Autodesk Fusion 360 part; units mm, degrees
(part 5 of 5)
sketch "Sketch7" plane through (0, 0, 13) normal (0, 0, -1) x (-1, 0, 0)
  line L0 (38.5, 121.5) -> (21.5, 121.5)
  line L1 (21.5, 121.5) -> (21.5, 138.5)
  line L2 (21.5, 138.5) -> (38.5, 138.5)
  line L3 (38.5, 138.5) -> (38.5, 121.5)
  line L4 (18.5, 121.5) -> (1.5, 121.5)
  line L5 (1.5, 121.5) -> (1.5, 138.5)
  line L6 (1.5, 138.5) -> (18.5, 138.5)
  line L7 (18.5, 138.5) -> (18.5, 121.5)
  line L8 (-1.5, 121.5) -> (-18.5, 121.5)
  line L9 (-18.5, 121.5) -> (-18.5, 138.5)
  line L10 (-18.5, 138.5) -> (-1.5, 138.5)
  line L11 (-1.5, 138.5) -> (-1.5, 121.5)
  line L12 (-21.5, 121.5) -> (-38.5, 121.5)
  line L13 (-38.5, 121.5) -> (-38.5, 138.5)
  line L14 (-38.5, 138.5) -> (-21.5, 138.5)
  line L15 (-21.5, 138.5) -> (-21.5, 121.5)
  line L16 (-41.5, 121.5) -> (-58.5, 121.5)
  line L17 (-58.5, 121.5) -> (-58.5, 138.5)
  line L18 (-58.5, 138.5) -> (-41.5, 138.5)
  line L19 (-41.5, 138.5) -> (-41.5, 121.5)
  line L20 (-61.5, 121.5) -> (-78.5, 121.5)
  line L21 (-78.5, 121.5) -> (-78.5, 138.5)
  line L22 (-78.5, 138.5) -> (-61.5, 138.5)
  line L23 (-61.5, 138.5) -> (-61.5, 121.5)
  line L24 (-81.5, 121.5) -> (-98.5, 121.5)
  line L25 (-98.5, 121.5) -> (-98.5, 138.5)
  line L26 (-98.5, 138.5) -> (-81.5, 138.5)
  line L27 (-81.5, 138.5) -> (-81.5, 121.5)
  line L28 (98.5, 141.5) -> (81.5, 141.5)
  line L29 (81.5, 141.5) -> (81.5, 158.5)
  line L30 (81.5, 158.5) -> (98.5, 158.5)
  line L31 (98.5, 158.5) -> (98.5, 141.5)
  line L32 (78.5, 141.5) -> (61.5, 141.5)
  line L33 (61.5, 141.5) -> (61.5, 158.5)
  line L34 (61.5, 158.5) -> (78.5, 158.5)
  line L35 (78.5, 158.5) -> (78.5, 141.5)
  line L36 (58.5, 141.5) -> (41.5, 141.5)
  line L37 (41.5, 141.5) -> (41.5, 158.5)
  line L38 (41.5, 158.5) -> (58.5, 158.5)
  line L39 (58.5, 158.5) -> (58.5, 141.5)
  line L40 (38.5, 141.5) -> (21.5, 141.5)
  line L41 (21.5, 141.5) -> (21.5, 158.5)
  line L42 (21.5, 158.5) -> (38.5, 158.5)
  line L43 (38.5, 158.5) -> (38.5, 141.5)
  line L44 (18.5, 141.5) -> (1.5, 141.5)
  line L45 (1.5, 141.5) -> (1.5, 158.5)
  line L46 (1.5, 158.5) -> (18.5, 158.5)
  line L47 (18.5, 158.5) -> (18.5, 141.5)
  line L48 (-1.5, 141.5) -> (-18.5, 141.5)
  line L49 (-18.5, 141.5) -> (-18.5, 158.5)
  line L50 (-18.5, 158.5) -> (-1.5, 158.5)
  line L51 (-1.5, 158.5) -> (-1.5, 141.5)
  line L52 (-21.5, 141.5) -> (-38.5, 141.5)
  line L53 (-38.5, 141.5) -> (-38.5, 158.5)
  line L54 (-38.5, 158.5) -> (-21.5, 158.5)
  line L55 (-21.5, 158.5) -> (-21.5, 141.5)
  line L56 (-41.5, 141.5) -> (-58.5, 141.5)
  line L57 (-58.5, 141.5) -> (-58.5, 158.5)
  line L58 (-58.5, 158.5) -> (-41.5, 158.5)
  line L59 (-41.5, 158.5) -> (-41.5, 141.5)
  line L60 (-61.5, 141.5) -> (-78.5, 141.5)
  line L61 (-78.5, 141.5) -> (-78.5, 158.5)
  line L62 (-78.5, 158.5) -> (-61.5, 158.5)
  line L63 (-61.5, 158.5) -> (-61.5, 141.5)
  line L64 (-81.5, 141.5) -> (-98.5, 141.5)
  line L65 (-98.5, 141.5) -> (-98.5, 158.5)
  line L66 (-98.5, 158.5) -> (-81.5, 158.5)
  line L67 (-81.5, 158.5) -> (-81.5, 141.5)
  line L68 (98.5, 161.5) -> (81.5, 161.5)
  line L69 (81.5, 161.5) -> (81.5, 178.5)
  line L70 (81.5, 178.5) -> (98.5, 178.5)
  line L71 (98.5, 178.5) -> (98.5, 161.5)
  line L72 (78.5, 161.5) -> (61.5, 161.5)
  line L73 (61.5, 161.5) -> (61.5, 178.5)
  line L74 (61.5, 178.5) -> (78.5, 178.5)
  line L75 (78.5, 178.5) -> (78.5, 161.5)
  line L76 (58.5, 161.5) -> (41.5, 161.5)
  line L77 (41.5, 161.5) -> (41.5, 178.5)
  line L78 (41.5, 178.5) -> (58.5, 178.5)
  line L79 (58.5, 178.5) -> (58.5, 161.5)
  line L80 (58.5, 121.5) -> (41.5, 121.5)
  line L81 (41.5, 121.5) -> (41.5, 138.5)
  line L82 (41.5, 138.5) -> (58.5, 138.5)
  line L83 (58.5, 138.5) -> (58.5, 121.5)
  line L84 (98.5, -98.5) -> (81.5, -98.5)
  line L85 (81.5, -98.5) -> (81.5, -81.5)
  line L86 (81.5, -81.5) -> (98.5, -81.5)
  line L87 (98.5, -81.5) -> (98.5, -98.5)
  line L88 (-1.5, -58.5) -> (-18.5, -58.5)
  line L89 (-18.5, -58.5) -> (-18.5, -41.5)
  line L90 (-18.5, -41.5) -> (-1.5, -41.5)
  line L91 (-1.5, -41.5) -> (-1.5, -58.5)
  line L92 (-81.5, -118.5) -> (-98.5, -118.5)
  line L93 (-98.5, -118.5) -> (-98.5, -101.5)
  line L94 (-98.5, -101.5) -> (-81.5, -101.5)
  line L95 (-81.5, -101.5) -> (-81.5, -118.5)
  line L96 (-61.5, -118.5) -> (-78.5, -118.5)
  line L97 (-78.5, -118.5) -> (-78.5, -101.5)
  line L98 (-78.5, -101.5) -> (-61.5, -101.5)
  line L99 (-61.5, -101.5) -> (-61.5, -118.5)
  line L100 (-41.5, -118.5) -> (-58.5, -118.5)
  line L101 (-58.5, -118.5) -> (-58.5, -101.5)
  line L102 (-58.5, -101.5) -> (-41.5, -101.5)
  line L103 (-41.5, -101.5) -> (-41.5, -118.5)
  line L104 (-21.5, -118.5) -> (-38.5, -118.5)
  line L105 (-38.5, -118.5) -> (-38.5, -101.5)
  line L106 (-38.5, -101.5) -> (-21.5, -101.5)
  line L107 (-21.5, -101.5) -> (-21.5, -118.5)
  line L108 (-1.5, -118.5) -> (-18.5, -118.5)
  line L109 (-18.5, -118.5) -> (-18.5, -101.5)
  line L110 (-18.5, -101.5) -> (-1.5, -101.5)
  line L111 (-1.5, -101.5) -> (-1.5, -118.5)
  line L112 (18.5, -118.5) -> (1.5, -118.5)
  line L113 (1.5, -118.5) -> (1.5, -101.5)
  line L114 (1.5, -101.5) -> (18.5, -101.5)
  line L115 (18.5, -101.5) -> (18.5, -118.5)
  line L116 (38.5, -118.5) -> (21.5, -118.5)
  line L117 (21.5, -118.5) -> (21.5, -101.5)
  line L118 (21.5, -101.5) -> (38.5, -101.5)
  line L119 (38.5, -101.5) -> (38.5, -118.5)
  line L120 (58.5, -118.5) -> (41.5, -118.5)
  line L121 (41.5, -118.5) -> (41.5, -101.5)
  line L122 (41.5, -101.5) -> (58.5, -101.5)
  line L123 (58.5, -101.5) -> (58.5, -118.5)
  line L124 (78.5, -118.5) -> (61.5, -118.5)
  line L125 (61.5, -118.5) -> (61.5, -101.5)
  line L126 (61.5, -101.5) -> (78.5, -101.5)
  line L127 (78.5, -101.5) -> (78.5, -118.5)
  line L128 (98.5, -118.5) -> (81.5, -118.5)
  line L129 (81.5, -118.5) -> (81.5, -101.5)
  line L130 (81.5, -101.5) -> (98.5, -101.5)
  line L131 (98.5, -101.5) -> (98.5, -118.5)
  line L132 (-81.5, -138.5) -> (-98.5, -138.5)
  line L133 (-98.5, -138.5) -> (-98.5, -121.5)
  line L134 (-98.5, -121.5) -> (-81.5, -121.5)
  line L135 (-81.5, -121.5) -> (-81.5, -138.5)
  line L136 (-61.5, -138.5) -> (-78.5, -138.5)
  line L137 (-78.5, -138.5) -> (-78.5, -121.5)
  line L138 (-78.5, -121.5) -> (-61.5, -121.5)
  line L139 (-61.5, -121.5) -> (-61.5, -138.5)
  line L140 (-41.5, -138.5) -> (-58.5, -138.5)
  line L141 (-58.5, -138.5) -> (-58.5, -121.5)
  line L142 (-58.5, -121.5) -> (-41.5, -121.5)
  line L143 (-41.5, -121.5) -> (-41.5, -138.5)
  line L144 (-21.5, -138.5) -> (-38.5, -138.5)
  line L145 (-38.5, -138.5) -> (-38.5, -121.5)
  line L146 (-38.5, -121.5) -> (-21.5, -121.5)
  line L147 (-21.5, -121.5) -> (-21.5, -138.5)
  line L148 (-1.5, -138.5) -> (-18.5, -138.5)
  line L149 (-18.5, -138.5) -> (-18.5, -121.5)
  line L150 (-18.5, -121.5) -> (-1.5, -121.5)
  line L151 (-1.5, -121.5) -> (-1.5, -138.5)
  line L152 (18.5, -138.5) -> (1.5, -138.5)
  line L153 (1.5, -138.5) -> (1.5, -121.5)
  line L154 (1.5, -121.5) -> (18.5, -121.5)
  line L155 (18.5, -121.5) -> (18.5, -138.5)
  line L156 (38.5, -138.5) -> (21.5, -138.5)
  line L157 (21.5, -138.5) -> (21.5, -121.5)
  line L158 (21.5, -121.5) -> (38.5, -121.5)
  line L159 (38.5, -121.5) -> (38.5, -138.5)
  line L160 (58.5, -138.5) -> (41.5, -138.5)
  line L161 (41.5, -138.5) -> (41.5, -121.5)
  line L162 (41.5, -121.5) -> (58.5, -121.5)
  line L163 (58.5, -121.5) -> (58.5, -138.5)
  line L164 (78.5, -138.5) -> (61.5, -138.5)
  line L165 (61.5, -138.5) -> (61.5, -121.5)
  line L166 (61.5, -121.5) -> (78.5, -121.5)
  line L167 (78.5, -121.5) -> (78.5, -138.5)
  line L168 (98.5, -138.5) -> (81.5, -138.5)
  line L169 (81.5, -138.5) -> (81.5, -121.5)
  line L170 (81.5, -121.5) -> (98.5, -121.5)
  line L171 (98.5, -121.5) -> (98.5, -138.5)
  line L172 (-81.5, -158.5) -> (-98.5, -158.5)
  line L173 (-98.5, -158.5) -> (-98.5, -141.5)
  line L174 (-98.5, -141.5) -> (-81.5, -141.5)
  line L175 (-81.5, -141.5) -> (-81.5, -158.5)
  line L176 (-61.5, -158.5) -> (-78.5, -158.5)
  line L177 (-78.5, -158.5) -> (-78.5, -141.5)
  line L178 (-78.5, -141.5) -> (-61.5, -141.5)
  line L179 (-61.5, -141.5) -> (-61.5, -158.5)
  line L180 (-41.5, -158.5) -> (-58.5, -158.5)
  line L181 (-58.5, -158.5) -> (-58.5, -141.5)
  line L182 (-58.5, -141.5) -> (-41.5, -141.5)
  line L183 (-41.5, -141.5) -> (-41.5, -158.5)
  line L184 (-21.5, -158.5) -> (-38.5, -158.5)
  line L185 (-38.5, -158.5) -> (-38.5, -141.5)
  line L186 (-38.5, -141.5) -> (-21.5, -141.5)
  line L187 (-21.5, -141.5) -> (-21.5, -158.5)
  line L188 (-1.5, -158.5) -> (-18.5, -158.5)
  line L189 (-18.5, -158.5) -> (-18.5, -141.5)
  line L190 (-18.5, -141.5) -> (-1.5, -141.5)
  line L191 (-1.5, -141.5) -> (-1.5, -158.5)
  line L192 (18.5, -158.5) -> (1.5, -158.5)
  line L193 (1.5, -158.5) -> (1.5, -141.5)
  line L194 (1.5, -141.5) -> (18.5, -141.5)
  line L195 (18.5, -141.5) -> (18.5, -158.5)
  line L196 (38.5, -158.5) -> (21.5, -158.5)
  line L197 (21.5, -158.5) -> (21.5, -141.5)
  line L198 (21.5, -141.5) -> (38.5, -141.5)
  line L199 (38.5, -141.5) -> (38.5, -158.5)
  line L200 (58.5, -158.5) -> (41.5, -158.5)
  line L201 (41.5, -158.5) -> (41.5, -141.5)
  line L202 (41.5, -141.5) -> (58.5, -141.5)
  line L203 (58.5, -141.5) -> (58.5, -158.5)
  line L204 (-41.5, -58.5) -> (-58.5, -58.5)
  line L205 (-58.5, -58.5) -> (-58.5, -41.5)
  line L206 (-58.5, -41.5) -> (-41.5, -41.5)
  line L207 (-41.5, -41.5) -> (-41.5, -58.5)
  line L208 (98.5, -201.5) -> (98.5, -218.5)
  line L209 (98.5, -218.5) -> (81.5, -218.5)
  line L210 (81.5, -218.5) -> (81.5, -201.5)
  line L211 (81.5, -201.5) -> (98.5, -201.5)
  line L212 (78.5, -218.5) -> (61.5, -218.5)
  line L213 (61.5, -218.5) -> (61.5, -201.5)
  line L214 (61.5, -201.5) -> (78.5, -201.5)
  line L215 (78.5, -201.5) -> (78.5, -218.5)
  line L216 (58.5, -218.5) -> (41.5, -218.5)
  line L217 (41.5, -218.5) -> (41.5, -201.5)
  line L218 (41.5, -201.5) -> (58.5, -201.5)
  line L219 (58.5, -201.5) -> (58.5, -218.5)
  line L220 (38.5, -218.5) -> (21.5, -218.5)
  line L221 (21.5, -218.5) -> (21.5, -201.5)
  line L222 (21.5, -201.5) -> (38.5, -201.5)
  line L223 (38.5, -201.5) -> (38.5, -218.5)
  line L224 (18.5, -218.5) -> (1.5, -218.5)
  line L225 (1.5, -218.5) -> (1.5, -201.5)
  line L226 (1.5, -201.5) -> (18.5, -201.5)
  line L227 (18.5, -201.5) -> (18.5, -218.5)
  line L228 (-1.5, -218.5) -> (-18.5, -218.5)
  line L229 (-18.5, -218.5) -> (-18.5, -201.5)
  line L230 (-18.5, -201.5) -> (-1.5, -201.5)
  line L231 (-1.5, -201.5) -> (-1.5, -218.5)
  line L232 (-21.5, -218.5) -> (-38.5, -218.5)
  line L233 (-38.5, -218.5) -> (-38.5, -201.5)
  line L234 (-38.5, -201.5) -> (-21.5, -201.5)
  line L235 (-21.5, -201.5) -> (-21.5, -218.5)
  line L236 (-41.5, -218.5) -> (-58.5, -218.5)
  line L237 (-58.5, -218.5) -> (-58.5, -201.5)
  line L238 (-58.5, -201.5) -> (-41.5, -201.5)
  line L239 (-41.5, -201.5) -> (-41.5, -218.5)
  line L240 (-61.5, -218.5) -> (-78.5, -218.5)
  line L241 (-78.5, -218.5) -> (-78.5, -201.5)
  line L242 (-78.5, -201.5) -> (-61.5, -201.5)
  line L243 (-61.5, -201.5) -> (-61.5, -218.5)
  line L244 (-81.5, -218.5) -> (-98.5, -218.5)
  line L245 (-98.5, -218.5) -> (-98.5, -201.5)
  line L246 (-98.5, -201.5) -> (-81.5, -201.5)
  line L247 (-81.5, -201.5) -> (-81.5, -218.5)
  line L248 (98.5, -198.5) -> (81.5, -198.5)
  line L249 (81.5, -198.5) -> (81.5, -181.5)
  line L250 (81.5, -181.5) -> (98.5, -181.5)
  line L251 (98.5, -181.5) -> (98.5, -198.5)
  line L252 (78.5, -198.5) -> (61.5, -198.5)
  line L253 (61.5, -198.5) -> (61.5, -181.5)
  line L254 (61.5, -181.5) -> (78.5, -181.5)
  line L255 (78.5, -181.5) -> (78.5, -198.5)
  line L256 (58.5, -198.5) -> (41.5, -198.5)
  line L257 (41.5, -198.5) -> (41.5, -181.5)
  line L258 (41.5, -181.5) -> (58.5, -181.5)
  line L259 (58.5, -181.5) -> (58.5, -198.5)
  line L260 (38.5, -198.5) -> (21.5, -198.5)
  line L261 (21.5, -198.5) -> (21.5, -181.5)
  line L262 (21.5, -181.5) -> (38.5, -181.5)
  line L263 (38.5, -181.5) -> (38.5, -198.5)
  line L264 (18.5, -198.5) -> (1.5, -198.5)
  line L265 (1.5, -198.5) -> (1.5, -181.5)
  line L266 (1.5, -181.5) -> (18.5, -181.5)
  line L267 (18.5, -181.5) -> (18.5, -198.5)
  line L268 (-1.5, -198.5) -> (-18.5, -198.5)
  line L269 (-18.5, -198.5) -> (-18.5, -181.5)
  line L270 (-18.5, -181.5) -> (-1.5, -181.5)
  line L271 (-1.5, -181.5) -> (-1.5, -198.5)
  line L272 (-21.5, -198.5) -> (-38.5, -198.5)
  line L273 (-38.5, -198.5) -> (-38.5, -181.5)
  line L274 (-38.5, -181.5) -> (-21.5, -181.5)
  line L275 (-21.5, -181.5) -> (-21.5, -198.5)
  line L276 (-41.5, -198.5) -> (-58.5, -198.5)
  line L277 (-58.5, -198.5) -> (-58.5, -181.5)
  line L278 (-58.5, -181.5) -> (-41.5, -181.5)
  line L279 (-41.5, -181.5) -> (-41.5, -198.5)
  line L280 (-61.5, -198.5) -> (-78.5, -198.5)
  line L281 (-78.5, -198.5) -> (-78.5, -181.5)
  line L282 (-78.5, -181.5) -> (-61.5, -181.5)
  line L283 (-61.5, -181.5) -> (-61.5, -198.5)
  line L284 (-81.5, -198.5) -> (-98.5, -198.5)
  line L285 (-98.5, -198.5) -> (-98.5, -181.5)
  line L286 (-98.5, -181.5) -> (-81.5, -181.5)
  line L287 (-81.5, -181.5) -> (-81.5, -198.5)
  line L288 (98.5, -178.5) -> (81.5, -178.5)
  line L289 (81.5, -178.5) -> (81.5, -161.5)
  line L290 (81.5, -161.5) -> (98.5, -161.5)
  line L291 (98.5, -161.5) -> (98.5, -178.5)
  line L292 (78.5, -178.5) -> (61.5, -178.5)
  line L293 (61.5, -178.5) -> (61.5, -161.5)
  line L294 (61.5, -161.5) -> (78.5, -161.5)
  line L295 (78.5, -161.5) -> (78.5, -178.5)
  line L296 (58.5, -178.5) -> (41.5, -178.5)
  line L297 (41.5, -178.5) -> (41.5, -161.5)
  line L298 (41.5, -161.5) -> (58.5, -161.5)
  line L299 (58.5, -161.5) -> (58.5, -178.5)
  line L300 (38.5, -178.5) -> (21.5, -178.5)
  line L301 (21.5, -178.5) -> (21.5, -161.5)
  line L302 (21.5, -161.5) -> (38.5, -161.5)
  line L303 (38.5, -161.5) -> (38.5, -178.5)
  line L304 (18.5, -178.5) -> (1.5, -178.5)
  line L305 (1.5, -178.5) -> (1.5, -161.5)
  line L306 (1.5, -161.5) -> (18.5, -161.5)
  line L307 (18.5, -161.5) -> (18.5, -178.5)
  line L308 (-1.5, -178.5) -> (-18.5, -178.5)
  line L309 (-18.5, -178.5) -> (-18.5, -161.5)
  line L310 (-18.5, -161.5) -> (-1.5, -161.5)
  line L311 (-1.5, -161.5) -> (-1.5, -178.5)
  line L312 (98.5, -158.5) -> (81.5, -158.5)
  line L313 (81.5, -158.5) -> (81.5, -141.5)
  line L314 (81.5, -141.5) -> (98.5, -141.5)
  line L315 (98.5, -141.5) -> (98.5, -158.5)
  line L316 (78.5, -158.5) -> (61.5, -158.5)
  line L317 (61.5, -158.5) -> (61.5, -141.5)
  line L318 (61.5, -141.5) -> (78.5, -141.5)
  line L319 (78.5, -141.5) -> (78.5, -158.5)
  line L320 (-81.5, -178.5) -> (-98.5, -178.5)
  line L321 (-98.5, -178.5) -> (-98.5, -161.5)
  line L322 (-98.5, -161.5) -> (-81.5, -161.5)
  line L323 (-81.5, -161.5) -> (-81.5, -178.5)
  line L324 (-61.5, -178.5) -> (-78.5, -178.5)
  line L325 (-78.5, -178.5) -> (-78.5, -161.5)
  line L326 (-78.5, -161.5) -> (-61.5, -161.5)
  line L327 (-61.5, -161.5) -> (-61.5, -178.5)
  line L328 (-41.5, -178.5) -> (-58.5, -178.5)
  line L329 (-58.5, -178.5) -> (-58.5, -161.5)
  line L330 (-58.5, -161.5) -> (-41.5, -161.5)
  line L331 (-41.5, -161.5) -> (-41.5, -178.5)
  line L332 (-21.5, -178.5) -> (-38.5, -178.5)
  line L333 (-38.5, -178.5) -> (-38.5, -161.5)
  line L334 (-38.5, -161.5) -> (-21.5, -161.5)
  line L335 (-21.5, -161.5) -> (-21.5, -178.5)
  line L336 (38.5, 161.5) -> (21.5, 161.5)
  line L337 (21.5, 161.5) -> (21.5, 178.5)
  line L338 (21.5, 178.5) -> (38.5, 178.5)
  line L339 (38.5, 178.5) -> (38.5, 161.5)
  line L340 (78.5, -98.5) -> (61.5, -98.5)
  line L341 (61.5, -98.5) -> (61.5, -81.5)
  line L342 (61.5, -81.5) -> (78.5, -81.5)
  line L343 (78.5, -81.5) -> (78.5, -98.5)
  line L344 (98.5, 121.5) -> (81.5, 121.5)
  line L345 (81.5, 121.5) -> (81.5, 138.5)
  line L346 (81.5, 138.5) -> (98.5, 138.5)
  line L347 (98.5, 138.5) -> (98.5, 121.5)
  line L348 (-81.5, 101.5) -> (-98.5, 101.5)
  line L349 (-98.5, 101.5) -> (-98.5, 118.5)
  line L350 (-98.5, 118.5) -> (-81.5, 118.5)
  line L351 (-81.5, 118.5) -> (-81.5, 101.5)
  line L352 (-61.5, 101.5) -> (-78.5, 101.5)
  line L353 (-78.5, 101.5) -> (-78.5, 118.5)
  line L354 (-78.5, 118.5) -> (-61.5, 118.5)
  line L355 (-61.5, 118.5) -> (-61.5, 101.5)
  line L356 (-41.5, 101.5) -> (-58.5, 101.5)
  line L357 (-58.5, 101.5) -> (-58.5, 118.5)
  line L358 (-58.5, 118.5) -> (-41.5, 118.5)
  line L359 (-41.5, 118.5) -> (-41.5, 101.5)
  line L360 (-21.5, 101.5) -> (-38.5, 101.5)
  line L361 (-38.5, 101.5) -> (-38.5, 118.5)
  line L362 (-38.5, 118.5) -> (-21.5, 118.5)
  line L363 (-21.5, 118.5) -> (-21.5, 101.5)
  line L364 (-1.5, 101.5) -> (-18.5, 101.5)
  line L365 (-18.5, 101.5) -> (-18.5, 118.5)
  line L366 (-18.5, 118.5) -> (-1.5, 118.5)
  line L367 (-1.5, 118.5) -> (-1.5, 101.5)
  line L368 (18.5, 101.5) -> (1.5, 101.5)
  line L369 (1.5, 101.5) -> (1.5, 118.5)
  line L370 (1.5, 118.5) -> (18.5, 118.5)
  line L371 (18.5, 118.5) -> (18.5, 101.5)
  line L372 (38.5, 101.5) -> (21.5, 101.5)
  line L373 (21.5, 101.5) -> (21.5, 118.5)
  line L374 (21.5, 118.5) -> (38.5, 118.5)
  line L375 (38.5, 118.5) -> (38.5, 101.5)
  line L376 (58.5, 101.5) -> (41.5, 101.5)
  line L377 (41.5, 101.5) -> (41.5, 118.5)
  line L378 (41.5, 118.5) -> (58.5, 118.5)
  line L379 (58.5, 118.5) -> (58.5, 101.5)
  line L380 (78.5, 101.5) -> (61.5, 101.5)
  line L381 (61.5, 101.5) -> (61.5, 118.5)
  line L382 (61.5, 118.5) -> (78.5, 118.5)
  line L383 (78.5, 118.5) -> (78.5, 101.5)
  line L384 (98.5, 101.5) -> (81.5, 101.5)
  line L385 (81.5, 101.5) -> (81.5, 118.5)
  line L386 (81.5, 118.5) -> (98.5, 118.5)
  line L387 (98.5, 118.5) -> (98.5, 101.5)
  line L388 (-81.5, 81.5) -> (-98.5, 81.5)
  line L389 (-98.5, 81.5) -> (-98.5, 98.5)
  line L390 (-98.5, 98.5) -> (-81.5, 98.5)
  line L391 (-81.5, 98.5) -> (-81.5, 81.5)
  line L392 (-61.5, 81.5) -> (-78.5, 81.5)
  line L393 (-78.5, 81.5) -> (-78.5, 98.5)
  line L394 (-78.5, 98.5) -> (-61.5, 98.5)
  line L395 (-61.5, 98.5) -> (-61.5, 81.5)
  line L396 (-41.5, 81.5) -> (-58.5, 81.5)
  line L397 (-58.5, 81.5) -> (-58.5, 98.5)
  line L398 (-58.5, 98.5) -> (-41.5, 98.5)
  line L399 (-41.5, 98.5) -> (-41.5, 81.5)
  line L400 (-21.5, 81.5) -> (-38.5, 81.5)
  line L401 (-38.5, 81.5) -> (-38.5, 98.5)
  line L402 (-38.5, 98.5) -> (-21.5, 98.5)
  line L403 (-21.5, 98.5) -> (-21.5, 81.5)
  line L404 (-1.5, 81.5) -> (-18.5, 81.5)
  line L405 (-18.5, 81.5) -> (-18.5, 98.5)
  line L406 (-18.5, 98.5) -> (-1.5, 98.5)
  line L407 (-1.5, 98.5) -> (-1.5, 81.5)
  line L408 (18.5, 81.5) -> (1.5, 81.5)
  line L409 (1.5, 81.5) -> (1.5, 98.5)
  line L410 (1.5, 98.5) -> (18.5, 98.5)
  line L411 (18.5, 98.5) -> (18.5, 81.5)
  line L412 (38.5, 81.5) -> (21.5, 81.5)
  line L413 (21.5, 81.5) -> (21.5, 98.5)
  line L414 (21.5, 98.5) -> (38.5, 98.5)
  line L415 (38.5, 98.5) -> (38.5, 81.5)
  line L416 (58.5, 81.5) -> (41.5, 81.5)
  line L417 (41.5, 81.5) -> (41.5, 98.5)
  line L418 (41.5, 98.5) -> (58.5, 98.5)
  line L419 (58.5, 98.5) -> (58.5, 81.5)
  line L420 (78.5, 81.5) -> (61.5, 81.5)
  line L421 (61.5, 81.5) -> (61.5, 98.5)
  line L422 (61.5, 98.5) -> (78.5, 98.5)
  line L423 (78.5, 98.5) -> (78.5, 81.5)
  line L424 (98.5, 81.5) -> (81.5, 81.5)
  line L425 (81.5, 81.5) -> (81.5, 98.5)
  line L426 (81.5, 98.5) -> (98.5, 98.5)
  line L427 (98.5, 98.5) -> (98.5, 81.5)
  line L428 (-81.5, 61.5) -> (-98.5, 61.5)
  line L429 (-98.5, 61.5) -> (-98.5, 78.5)
  line L430 (-98.5, 78.5) -> (-81.5, 78.5)
  line L431 (-81.5, 78.5) -> (-81.5, 61.5)
  line L432 (-61.5, 61.5) -> (-78.5, 61.5)
  line L433 (-78.5, 61.5) -> (-78.5, 78.5)
  line L434 (-78.5, 78.5) -> (-61.5, 78.5)
  line L435 (-61.5, 78.5) -> (-61.5, 61.5)
  line L436 (-41.5, 61.5) -> (-58.5, 61.5)
  line L437 (-58.5, 61.5) -> (-58.5, 78.5)
  line L438 (-58.5, 78.5) -> (-41.5, 78.5)
  line L439 (-41.5, 78.5) -> (-41.5, 61.5)
  line L440 (-21.5, 61.5) -> (-38.5, 61.5)
  line L441 (-38.5, 61.5) -> (-38.5, 78.5)
  line L442 (-38.5, 78.5) -> (-21.5, 78.5)
  line L443 (-21.5, 78.5) -> (-21.5, 61.5)
  line L444 (-1.5, 61.5) -> (-18.5, 61.5)
  line L445 (-18.5, 61.5) -> (-18.5, 78.5)
  line L446 (-18.5, 78.5) -> (-1.5, 78.5)
  line L447 (-1.5, 78.5) -> (-1.5, 61.5)
  line L448 (18.5, 61.5) -> (1.5, 61.5)
  line L449 (1.5, 61.5) -> (1.5, 78.5)
  line L450 (1.5, 78.5) -> (18.5, 78.5)
  line L451 (18.5, 78.5) -> (18.5, 61.5)
  line L452 (38.5, 61.5) -> (21.5, 61.5)
  line L453 (21.5, 61.5) -> (21.5, 78.5)
  line L454 (21.5, 78.5) -> (38.5, 78.5)
  line L455 (38.5, 78.5) -> (38.5, 61.5)
  line L456 (58.5, 61.5) -> (41.5, 61.5)
  line L457 (41.5, 61.5) -> (41.5, 78.5)
  line L458 (41.5, 78.5) -> (58.5, 78.5)
  line L459 (58.5, 78.5) -> (58.5, 61.5)
  line L460 (78.5, 61.5) -> (61.5, 61.5)
  line L461 (61.5, 61.5) -> (61.5, 78.5)
  line L462 (61.5, 78.5) -> (78.5, 78.5)
  line L463 (78.5, 78.5) -> (78.5, 61.5)
  line L464 (98.5, 61.5) -> (81.5, 61.5)
  line L465 (81.5, 61.5) -> (81.5, 78.5)
  line L466 (81.5, 78.5) -> (98.5, 78.5)
  line L467 (98.5, 78.5) -> (98.5, 61.5)
  line L468 (-81.5, 41.5) -> (-98.5, 41.5)
  line L469 (-98.5, 41.5) -> (-98.5, 58.5)
  line L470 (-98.5, 58.5) -> (-81.5, 58.5)
  line L471 (-81.5, 58.5) -> (-81.5, 41.5)
  line L472 (-61.5, 41.5) -> (-78.5, 41.5)
  line L473 (-78.5, 41.5) -> (-78.5, 58.5)
  line L474 (-78.5, 58.5) -> (-61.5, 58.5)
  line L475 (-61.5, 58.5) -> (-61.5, 41.5)
  line L476 (-41.5, 41.5) -> (-58.5, 41.5)
  line L477 (-58.5, 41.5) -> (-58.5, 58.5)
  line L478 (-58.5, 58.5) -> (-41.5, 58.5)
  line L479 (-41.5, 58.5) -> (-41.5, 41.5)
  line L480 (-21.5, 41.5) -> (-38.5, 41.5)
  line L481 (-38.5, 41.5) -> (-38.5, 58.5)
  line L482 (-38.5, 58.5) -> (-21.5, 58.5)
  line L483 (-21.5, 58.5) -> (-21.5, 41.5)
  line L484 (-1.5, 41.5) -> (-18.5, 41.5)
  line L485 (-18.5, 41.5) -> (-18.5, 58.5)
  line L486 (-18.5, 58.5) -> (-1.5, 58.5)
  line L487 (-1.5, 58.5) -> (-1.5, 41.5)
  line L488 (18.5, 41.5) -> (1.5, 41.5)
  line L489 (1.5, 41.5) -> (1.5, 58.5)
  line L490 (1.5, 58.5) -> (18.5, 58.5)
  line L491 (18.5, 58.5) -> (18.5, 41.5)
  line L492 (38.5, 41.5) -> (21.5, 41.5)
  line L493 (21.5, 41.5) -> (21.5, 58.5)
  line L494 (21.5, 58.5) -> (38.5, 58.5)
  line L495 (38.5, 58.5) -> (38.5, 41.5)
  line L496 (58.5, 41.5) -> (41.5, 41.5)
  line L497 (41.5, 41.5) -> (41.5, 58.5)
  line L498 (41.5, 58.5) -> (58.5, 58.5)
  line L499 (58.5, 58.5) -> (58.5, 41.5)
  line L500 (78.5, 41.5) -> (61.5, 41.5)
  line L501 (61.5, 41.5) -> (61.5, 58.5)
  line L502 (61.5, 58.5) -> (78.5, 58.5)
  line L503 (78.5, 58.5) -> (78.5, 41.5)
  line L504 (98.5, 41.5) -> (81.5, 41.5)
  line L505 (81.5, 41.5) -> (81.5, 58.5)
  line L506 (81.5, 58.5) -> (98.5, 58.5)
  line L507 (98.5, 58.5) -> (98.5, 41.5)
  line L508 (-81.5, 21.5) -> (-98.5, 21.5)
  line L509 (-98.5, 21.5) -> (-98.5, 38.5)
  line L510 (-98.5, 38.5) -> (-81.5, 38.5)
  line L511 (-81.5, 38.5) -> (-81.5, 21.5)
  line L512 (-61.5, 21.5) -> (-78.5, 21.5)
  line L513 (-78.5, 21.5) -> (-78.5, 38.5)
  line L514 (-78.5, 38.5) -> (-61.5, 38.5)
  line L515 (-61.5, 38.5) -> (-61.5, 21.5)
  line L516 (-41.5, 21.5) -> (-58.5, 21.5)
  line L517 (-58.5, 21.5) -> (-58.5, 38.5)
  line L518 (-58.5, 38.5) -> (-41.5, 38.5)
  line L519 (-41.5, 38.5) -> (-41.5, 21.5)
  line L520 (-21.5, 21.5) -> (-38.5, 21.5)
  line L521 (-38.5, 21.5) -> (-38.5, 38.5)
  line L522 (-38.5, 38.5) -> (-21.5, 38.5)
  line L523 (-21.5, 38.5) -> (-21.5, 21.5)
  line L524 (-1.5, 21.5) -> (-18.5, 21.5)
  line L525 (-18.5, 21.5) -> (-18.5, 38.5)
  line L526 (-18.5, 38.5) -> (-1.5, 38.5)
  line L527 (-1.5, 38.5) -> (-1.5, 21.5)
  line L528 (18.5, 21.5) -> (1.5, 21.5)
  line L529 (1.5, 21.5) -> (1.5, 38.5)
  line L530 (1.5, 38.5) -> (18.5, 38.5)
  line L531 (18.5, 38.5) -> (18.5, 21.5)
  line L532 (38.5, 21.5) -> (21.5, 21.5)
  line L533 (21.5, 21.5) -> (21.5, 38.5)
  line L534 (21.5, 38.5) -> (38.5, 38.5)
  line L535 (38.5, 38.5) -> (38.5, 21.5)
  line L536 (58.5, 21.5) -> (41.5, 21.5)
  line L537 (41.5, 21.5) -> (41.5, 38.5)
  line L538 (41.5, 38.5) -> (58.5, 38.5)
  line L539 (58.5, 38.5) -> (58.5, 21.5)
  line L540 (78.5, 21.5) -> (61.5, 21.5)
  line L541 (61.5, 21.5) -> (61.5, 38.5)
  line L542 (61.5, 38.5) -> (78.5, 38.5)
  line L543 (78.5, 38.5) -> (78.5, 21.5)
  line L544 (98.5, 21.5) -> (81.5, 21.5)
  line L545 (81.5, 21.5) -> (81.5, 38.5)
  line L546 (81.5, 38.5) -> (98.5, 38.5)
  line L547 (98.5, 38.5) -> (98.5, 21.5)
  line L548 (-81.5, 1.5) -> (-98.5, 1.5)
  line L549 (-98.5, 1.5) -> (-98.5, 18.5)
  line L550 (-98.5, 18.5) -> (-81.5, 18.5)
  line L551 (-81.5, 18.5) -> (-81.5, 1.5)
  line L552 (-61.5, 1.5) -> (-78.5, 1.5)
  line L553 (-78.5, 1.5) -> (-78.5, 18.5)
  line L554 (-78.5, 18.5) -> (-61.5, 18.5)
  line L555 (-61.5, 18.5) -> (-61.5, 1.5)
  line L556 (-41.5, 1.5) -> (-58.5, 1.5)
  line L557 (-58.5, 1.5) -> (-58.5, 18.5)
  line L558 (-58.5, 18.5) -> (-41.5, 18.5)
  line L559 (-41.5, 18.5) -> (-41.5, 1.5)
  line L560 (-21.5, 1.5) -> (-38.5, 1.5)
  line L561 (-38.5, 1.5) -> (-38.5, 18.5)
  line L562 (-38.5, 18.5) -> (-21.5, 18.5)
  line L563 (-21.5, 18.5) -> (-21.5, 1.5)
  line L564 (-1.5, 1.5) -> (-18.5, 1.5)
  line L565 (-18.5, 1.5) -> (-18.5, 18.5)
  line L566 (-18.5, 18.5) -> (-1.5, 18.5)
  line L567 (-1.5, 18.5) -> (-1.5, 1.5)
  line L568 (18.5, 1.5) -> (1.5, 1.5)
  line L569 (1.5, 1.5) -> (1.5, 18.5)
  line L570 (1.5, 18.5) -> (18.5, 18.5)
  line L571 (18.5, 18.5) -> (18.5, 1.5)
  line L572 (38.5, 1.5) -> (21.5, 1.5)
  line L573 (21.5, 1.5) -> (21.5, 18.5)
  line L574 (21.5, 18.5) -> (38.5, 18.5)
  line L575 (38.5, 18.5) -> (38.5, 1.5)
  line L576 (58.5, 1.5) -> (41.5, 1.5)
  line L577 (41.5, 1.5) -> (41.5, 18.5)
  line L578 (41.5, 18.5) -> (58.5, 18.5)
  line L579 (58.5, 18.5) -> (58.5, 1.5)
  line L580 (78.5, 1.5) -> (61.5, 1.5)
  line L581 (61.5, 1.5) -> (61.5, 18.5)
  line L582 (61.5, 18.5) -> (78.5, 18.5)
  line L583 (78.5, 18.5) -> (78.5, 1.5)
  line L584 (98.5, 1.5) -> (81.5, 1.5)
  line L585 (81.5, 1.5) -> (81.5, 18.5)
  line L586 (81.5, 18.5) -> (98.5, 18.5)
  line L587 (98.5, 18.5) -> (98.5, 1.5)
  line L588 (-81.5, -18.5) -> (-98.5, -18.5)
  line L589 (-98.5, -18.5) -> (-98.5, -1.5)
  line L590 (-98.5, -1.5) -> (-81.5, -1.5)
  line L591 (-81.5, -1.5) -> (-81.5, -18.5)
  line L592 (-61.5, -18.5) -> (-78.5, -18.5)
  line L593 (-78.5, -18.5) -> (-78.5, -1.5)
  line L594 (-78.5, -1.5) -> (-61.5, -1.5)
  line L595 (-61.5, -1.5) -> (-61.5, -18.5)
  line L596 (-41.5, -18.5) -> (-58.5, -18.5)
  line L597 (-58.5, -18.5) -> (-58.5, -1.5)
  line L598 (-58.5, -1.5) -> (-41.5, -1.5)
  line L599 (-41.5, -1.5) -> (-41.5, -18.5)
  line L600 (-21.5, -18.5) -> (-38.5, -18.5)
  line L601 (-38.5, -18.5) -> (-38.5, -1.5)
  line L602 (-38.5, -1.5) -> (-21.5, -1.5)
  line L603 (-21.5, -1.5) -> (-21.5, -18.5)
  line L604 (-1.5, -18.5) -> (-18.5, -18.5)
  line L605 (-18.5, -18.5) -> (-18.5, -1.5)
  line L606 (-18.5, -1.5) -> (-1.5, -1.5)
  line L607 (-1.5, -1.5) -> (-1.5, -18.5)
  line L608 (18.5, -18.5) -> (1.5, -18.5)
  line L609 (1.5, -18.5) -> (1.5, -1.5)
  line L610 (1.5, -1.5) -> (18.5, -1.5)
  line L611 (18.5, -1.5) -> (18.5, -18.5)
  line L612 (38.5, -18.5) -> (21.5, -18.5)
  line L613 (21.5, -18.5) -> (21.5, -1.5)
  line L614 (21.5, -1.5) -> (38.5, -1.5)
  line L615 (38.5, -1.5) -> (38.5, -18.5)
  line L616 (58.5, -18.5) -> (41.5, -18.5)
  line L617 (41.5, -18.5) -> (41.5, -1.5)
  line L618 (41.5, -1.5) -> (58.5, -1.5)
  line L619 (58.5, -1.5) -> (58.5, -18.5)
  line L620 (78.5, -18.5) -> (61.5, -18.5)
  line L621 (61.5, -18.5) -> (61.5, -1.5)
  line L622 (61.5, -1.5) -> (78.5, -1.5)
  line L623 (78.5, -1.5) -> (78.5, -18.5)
  line L624 (98.5, -18.5) -> (81.5, -18.5)
  line L625 (81.5, -18.5) -> (81.5, -1.5)
  line L626 (81.5, -1.5) -> (98.5, -1.5)
  line L627 (98.5, -1.5) -> (98.5, -18.5)
  line L628 (-81.5, -38.5) -> (-98.5, -38.5)
  line L629 (-98.5, -38.5) -> (-98.5, -21.5)
  line L630 (-98.5, -21.5) -> (-81.5, -21.5)
  line L631 (-81.5, -21.5) -> (-81.5, -38.5)
  line L632 (-61.5, -38.5) -> (-78.5, -38.5)
  line L633 (-78.5, -38.5) -> (-78.5, -21.5)
  line L634 (-78.5, -21.5) -> (-61.5, -21.5)
  line L635 (-61.5, -21.5) -> (-61.5, -38.5)
  line L636 (-41.5, -38.5) -> (-58.5, -38.5)
  line L637 (-58.5, -38.5) -> (-58.5, -21.5)
  line L638 (-58.5, -21.5) -> (-41.5, -21.5)
  line L639 (-41.5, -21.5) -> (-41.5, -38.5)
  line L640 (-21.5, -38.5) -> (-38.5, -38.5)
  line L641 (-38.5, -38.5) -> (-38.5, -21.5)
  line L642 (-38.5, -21.5) -> (-21.5, -21.5)
  line L643 (-21.5, -21.5) -> (-21.5, -38.5)
  line L644 (-1.5, -38.5) -> (-18.5, -38.5)
  line L645 (-18.5, -38.5) -> (-18.5, -21.5)
  line L646 (-18.5, -21.5) -> (-1.5, -21.5)
  line L647 (-1.5, -21.5) -> (-1.5, -38.5)
  line L648 (18.5, -38.5) -> (1.5, -38.5)
  line L649 (1.5, -38.5) -> (1.5, -21.5)
  line L650 (1.5, -21.5) -> (18.5, -21.5)
  line L651 (18.5, -21.5) -> (18.5, -38.5)
  line L652 (38.5, -38.5) -> (21.5, -38.5)
  line L653 (21.5, -38.5) -> (21.5, -21.5)
  line L654 (21.5, -21.5) -> (38.5, -21.5)
  line L655 (38.5, -21.5) -> (38.5, -38.5)
  line L656 (58.5, -38.5) -> (41.5, -38.5)
  line L657 (41.5, -38.5) -> (41.5, -21.5)
  line L658 (41.5, -21.5) -> (58.5, -21.5)
  line L659 (58.5, -21.5) -> (58.5, -38.5)
  line L660 (78.5, -38.5) -> (61.5, -38.5)
  line L661 (61.5, -38.5) -> (61.5, -21.5)
  line L662 (61.5, -21.5) -> (78.5, -21.5)
  line L663 (78.5, -21.5) -> (78.5, -38.5)
  line L664 (98.5, -38.5) -> (81.5, -38.5)
  line L665 (81.5, -38.5) -> (81.5, -21.5)
  line L666 (81.5, -21.5) -> (98.5, -21.5)
  line L667 (98.5, -21.5) -> (98.5, -38.5)
  line L668 (-81.5, -58.5) -> (-98.5, -58.5)
  line L669 (-98.5, -58.5) -> (-98.5, -41.5)
  line L670 (-98.5, -41.5) -> (-81.5, -41.5)
  line L671 (-81.5, -41.5) -> (-81.5, -58.5)
  line L672 (-61.5, -58.5) -> (-78.5, -58.5)
  line L673 (-78.5, -58.5) -> (-78.5, -41.5)
  line L674 (-78.5, -41.5) -> (-61.5, -41.5)
  line L675 (-61.5, -41.5) -> (-61.5, -58.5)
  line L676 (-81.5, 201.5) -> (-98.5, 201.5)
  line L677 (-98.5, 201.5) -> (-98.5, 218.5)
  line L678 (-98.5, 218.5) -> (-81.5, 218.5)
  line L679 (-81.5, 218.5) -> (-81.5, 201.5)
  line L680 (-61.5, 201.5) -> (-78.5, 201.5)
  line L681 (-78.5, 201.5) -> (-78.5, 218.5)
  line L682 (-78.5, 218.5) -> (-61.5, 218.5)
  line L683 (-61.5, 218.5) -> (-61.5, 201.5)
  line L684 (-41.5, 201.5) -> (-58.5, 201.5)
  line L685 (-58.5, 201.5) -> (-58.5, 218.5)
  line L686 (-58.5, 218.5) -> (-41.5, 218.5)
  line L687 (-41.5, 218.5) -> (-41.5, 201.5)
  line L688 (-21.5, 201.5) -> (-38.5, 201.5)
  line L689 (-38.5, 201.5) -> (-38.5, 218.5)
  line L690 (-38.5, 218.5) -> (-21.5, 218.5)
  line L691 (-21.5, 218.5) -> (-21.5, 201.5)
  line L692 (-1.5, 201.5) -> (-18.5, 201.5)
  line L693 (-18.5, 201.5) -> (-18.5, 218.5)
  line L694 (-18.5, 218.5) -> (-1.5, 218.5)
  line L695 (-1.5, 218.5) -> (-1.5, 201.5)
  line L696 (18.5, 201.5) -> (1.5, 201.5)
  line L697 (1.5, 201.5) -> (1.5, 218.5)
  line L698 (1.5, 218.5) -> (18.5, 218.5)
  line L699 (18.5, 218.5) -> (18.5, 201.5)
  line L700 (38.5, 201.5) -> (21.5, 201.5)
  line L701 (21.5, 201.5) -> (21.5, 218.5)
  line L702 (21.5, 218.5) -> (38.5, 218.5)
  line L703 (38.5, 218.5) -> (38.5, 201.5)
  line L704 (58.5, 201.5) -> (41.5, 201.5)
  line L705 (41.5, 201.5) -> (41.5, 218.5)
  line L706 (41.5, 218.5) -> (58.5, 218.5)
  line L707 (58.5, 218.5) -> (58.5, 201.5)
  line L708 (78.5, 201.5) -> (61.5, 201.5)
  line L709 (61.5, 201.5) -> (61.5, 218.5)
  line L710 (61.5, 218.5) -> (78.5, 218.5)
  line L711 (78.5, 218.5) -> (78.5, 201.5)
  line L712 (98.5, 201.5) -> (81.5, 201.5)
  line L713 (81.5, 201.5) -> (81.5, 218.5)
  line L714 (81.5, 218.5) -> (98.5, 218.5)
  line L715 (98.5, 218.5) -> (98.5, 201.5)
  line L716 (-81.5, 181.5) -> (-98.5, 181.5)
  line L717 (-98.5, 181.5) -> (-98.5, 198.5)
  line L718 (-98.5, 198.5) -> (-81.5, 198.5)
  line L719 (-81.5, 198.5) -> (-81.5, 181.5)
  line L720 (-61.5, 181.5) -> (-78.5, 181.5)
  line L721 (-78.5, 181.5) -> (-78.5, 198.5)
  line L722 (-78.5, 198.5) -> (-61.5, 198.5)
  line L723 (-61.5, 198.5) -> (-61.5, 181.5)
  line L724 (-41.5, 181.5) -> (-58.5, 181.5)
  line L725 (-58.5, 181.5) -> (-58.5, 198.5)
  line L726 (-58.5, 198.5) -> (-41.5, 198.5)
  line L727 (-41.5, 198.5) -> (-41.5, 181.5)
  line L728 (-21.5, 181.5) -> (-38.5, 181.5)
  line L729 (-38.5, 181.5) -> (-38.5, 198.5)
  line L730 (-38.5, 198.5) -> (-21.5, 198.5)
  line L731 (-21.5, 198.5) -> (-21.5, 181.5)
  line L732 (-1.5, 181.5) -> (-18.5, 181.5)
  line L733 (-18.5, 181.5) -> (-18.5, 198.5)
  line L734 (-18.5, 198.5) -> (-1.5, 198.5)
  line L735 (-1.5, 198.5) -> (-1.5, 181.5)
  line L736 (18.5, 181.5) -> (1.5, 181.5)
  line L737 (1.5, 181.5) -> (1.5, 198.5)
  line L738 (1.5, 198.5) -> (18.5, 198.5)
  line L739 (18.5, 198.5) -> (18.5, 181.5)
  line L740 (38.5, 181.5) -> (21.5, 181.5)
  line L741 (21.5, 181.5) -> (21.5, 198.5)
  line L742 (21.5, 198.5) -> (38.5, 198.5)
  line L743 (38.5, 198.5) -> (38.5, 181.5)
  line L744 (58.5, 181.5) -> (41.5, 181.5)
  line L745 (41.5, 181.5) -> (41.5, 198.5)
  line L746 (41.5, 198.5) -> (58.5, 198.5)
  line L747 (58.5, 198.5) -> (58.5, 181.5)
  line L748 (78.5, 181.5) -> (61.5, 181.5)
  line L749 (61.5, 181.5) -> (61.5, 198.5)
  line L750 (61.5, 198.5) -> (78.5, 198.5)
  line L751 (78.5, 198.5) -> (78.5, 181.5)
  line L752 (98.5, 181.5) -> (81.5, 181.5)
  line L753 (81.5, 181.5) -> (81.5, 198.5)
  line L754 (81.5, 198.5) -> (98.5, 198.5)
  line L755 (98.5, 198.5) -> (98.5, 181.5)
  line L756 (-81.5, 161.5) -> (-98.5, 161.5)
  line L757 (-98.5, 161.5) -> (-98.5, 178.5)
  line L758 (-98.5, 178.5) -> (-81.5, 178.5)
  line L759 (-81.5, 178.5) -> (-81.5, 161.5)
  line L760 (-61.5, 161.5) -> (-78.5, 161.5)
  line L761 (-78.5, 161.5) -> (-78.5, 178.5)
  line L762 (-78.5, 178.5) -> (-61.5, 178.5)
  line L763 (-61.5, 178.5) -> (-61.5, 161.5)
  line L764 (-41.5, 161.5) -> (-58.5, 161.5)
  line L765 (-58.5, 161.5) -> (-58.5, 178.5)
  line L766 (-58.5, 178.5) -> (-41.5, 178.5)
  line L767 (-41.5, 178.5) -> (-41.5, 161.5)
  line L768 (-21.5, 161.5) -> (-38.5, 161.5)
  line L769 (-38.5, 161.5) -> (-38.5, 178.5)
  line L770 (-38.5, 178.5) -> (-21.5, 178.5)
  line L771 (-21.5, 178.5) -> (-21.5, 161.5)
  line L772 (-1.5, 161.5) -> (-18.5, 161.5)
  line L773 (-18.5, 161.5) -> (-18.5, 178.5)
  line L774 (-18.5, 178.5) -> (-1.5, 178.5)
  line L775 (-1.5, 178.5) -> (-1.5, 161.5)
  line L776 (18.5, 161.5) -> (1.5, 161.5)
  line L777 (1.5, 161.5) -> (1.5, 178.5)
  line L778 (1.5, 178.5) -> (18.5, 178.5)
  line L779 (18.5, 178.5) -> (18.5, 161.5)
  line L780 (78.5, 121.5) -> (61.5, 121.5)
  line L781 (61.5, 121.5) -> (61.5, 138.5)
  line L782 (61.5, 138.5) -> (78.5, 138.5)
  line L783 (78.5, 138.5) -> (78.5, 121.5)
  line L784 (-21.5, -58.5) -> (-38.5, -58.5)
  line L785 (-38.5, -58.5) -> (-38.5, -41.5)
  line L786 (-38.5, -41.5) -> (-21.5, -41.5)
  line L787 (-21.5, -41.5) -> (-21.5, -58.5)
  line L788 (18.5, -58.5) -> (1.5, -58.5)
  line L789 (1.5, -58.5) -> (1.5, -41.5)
  line L790 (1.5, -41.5) -> (18.5, -41.5)
  line L791 (18.5, -41.5) -> (18.5, -58.5)
  line L792 (38.5, -58.5) -> (21.5, -58.5)
  line L793 (21.5, -58.5) -> (21.5, -41.5)
  line L794 (21.5, -41.5) -> (38.5, -41.5)
  line L795 (38.5, -41.5) -> (38.5, -58.5)
  line L796 (58.5, -58.5) -> (41.5, -58.5)
  line L797 (41.5, -58.5) -> (41.5, -41.5)
  line L798 (41.5, -41.5) -> (58.5, -41.5)
  line L799 (58.5, -41.5) -> (58.5, -58.5)
  line L800 (78.5, -58.5) -> (61.5, -58.5)
  line L801 (61.5, -58.5) -> (61.5, -41.5)
  line L802 (61.5, -41.5) -> (78.5, -41.5)
  line L803 (78.5, -41.5) -> (78.5, -58.5)
  line L804 (98.5, -58.5) -> (81.5, -58.5)
  line L805 (81.5, -58.5) -> (81.5, -41.5)
  line L806 (81.5, -41.5) -> (98.5, -41.5)
  line L807 (98.5, -41.5) -> (98.5, -58.5)
  line L808 (-81.5, -78.5) -> (-98.5, -78.5)
  line L809 (-98.5, -78.5) -> (-98.5, -61.5)
  line L810 (-98.5, -61.5) -> (-81.5, -61.5)
  line L811 (-81.5, -61.5) -> (-81.5, -78.5)
  line L812 (-61.5, -78.5) -> (-78.5, -78.5)
  line L813 (-78.5, -78.5) -> (-78.5, -61.5)
  line L814 (-78.5, -61.5) -> (-61.5, -61.5)
  line L815 (-61.5, -61.5) -> (-61.5, -78.5)
  line L816 (-41.5, -78.5) -> (-58.5, -78.5)
  line L817 (-58.5, -78.5) -> (-58.5, -61.5)
  line L818 (-58.5, -61.5) -> (-41.5, -61.5)
  line L819 (-41.5, -61.5) -> (-41.5, -78.5)
  line L820 (-21.5, -78.5) -> (-38.5, -78.5)
  line L821 (-38.5, -78.5) -> (-38.5, -61.5)
  line L822 (-38.5, -61.5) -> (-21.5, -61.5)
  line L823 (-21.5, -61.5) -> (-21.5, -78.5)
  line L824 (-1.5, -78.5) -> (-18.5, -78.5)
  line L825 (-18.5, -78.5) -> (-18.5, -61.5)
  line L826 (-18.5, -61.5) -> (-1.5, -61.5)
  line L827 (-1.5, -61.5) -> (-1.5, -78.5)
  line L828 (18.5, -78.5) -> (1.5, -78.5)
  line L829 (1.5, -78.5) -> (1.5, -61.5)
  line L830 (1.5, -61.5) -> (18.5, -61.5)
  line L831 (18.5, -61.5) -> (18.5, -78.5)
  line L832 (38.5, -78.5) -> (21.5, -78.5)
  line L833 (21.5, -78.5) -> (21.5, -61.5)
  line L834 (21.5, -61.5) -> (38.5, -61.5)
  line L835 (38.5, -61.5) -> (38.5, -78.5)
  line L836 (58.5, -78.5) -> (41.5, -78.5)
  line L837 (41.5, -78.5) -> (41.5, -61.5)
  line L838 (41.5, -61.5) -> (58.5, -61.5)
  line L839 (58.5, -61.5) -> (58.5, -78.5)
  line L840 (78.5, -78.5) -> (61.5, -78.5)
  line L841 (61.5, -78.5) -> (61.5, -61.5)
  line L842 (61.5, -61.5) -> (78.5, -61.5)
  line L843 (78.5, -61.5) -> (78.5, -78.5)
  line L844 (98.5, -78.5) -> (81.5, -78.5)
  line L845 (81.5, -78.5) -> (81.5, -61.5)
  line L846 (81.5, -61.5) -> (98.5, -61.5)
  line L847 (98.5, -61.5) -> (98.5, -78.5)
  line L848 (-81.5, -98.5) -> (-98.5, -98.5)
  line L849 (-98.5, -98.5) -> (-98.5, -81.5)
  line L850 (-98.5, -81.5) -> (-81.5, -81.5)
  line L851 (-81.5, -81.5) -> (-81.5, -98.5)
  line L852 (-61.5, -98.5) -> (-78.5, -98.5)
  line L853 (-78.5, -98.5) -> (-78.5, -81.5)
  line L854 (-78.5, -81.5) -> (-61.5, -81.5)
  line L855 (-61.5, -81.5) -> (-61.5, -98.5)
  line L856 (-41.5, -98.5) -> (-58.5, -98.5)
  line L857 (-58.5, -98.5) -> (-58.5, -81.5)
  line L858 (-58.5, -81.5) -> (-41.5, -81.5)
  line L859 (-41.5, -81.5) -> (-41.5, -98.5)
  line L860 (-21.5, -98.5) -> (-38.5, -98.5)
  line L861 (-38.5, -98.5) -> (-38.5, -81.5)
  line L862 (-38.5, -81.5) -> (-21.5, -81.5)
  line L863 (-21.5, -81.5) -> (-21.5, -98.5)
  line L864 (-1.5, -98.5) -> (-18.5, -98.5)
  line L865 (-18.5, -98.5) -> (-18.5, -81.5)
  line L866 (-18.5, -81.5) -> (-1.5, -81.5)
  line L867 (-1.5, -81.5) -> (-1.5, -98.5)
  line L868 (18.5, -98.5) -> (1.5, -98.5)
  line L869 (1.5, -98.5) -> (1.5, -81.5)
  line L870 (1.5, -81.5) -> (18.5, -81.5)
  line L871 (18.5, -81.5) -> (18.5, -98.5)
  line L872 (38.5, -98.5) -> (21.5, -98.5)
  line L873 (21.5, -98.5) -> (21.5, -81.5)
  line L874 (21.5, -81.5) -> (38.5, -81.5)
  line L875 (38.5, -81.5) -> (38.5, -98.5)
  line L876 (58.5, -98.5) -> (41.5, -98.5)
  line L877 (41.5, -98.5) -> (41.5, -81.5)
  line L878 (41.5, -81.5) -> (58.5, -81.5)
  line L879 (58.5, -81.5) -> (58.5, -98.5)
  line L880 (-105, -220) -> (105, -220)
  line L881 (105, -220) -> (105, 220)
  line L882 (105, 220) -> (-105, 220)
  line L883 (-105, 220) -> (-105, -220)
  line L884 (98.5, 218.5) -> (98.5, 220)
  line L885 (98.5, 220) -> (100, 220)
  line L886 (100, 220) -> (100, -220)
  line L887 (-98.5, -218.5) -> (-98.5, -220)
  line L888 (-98.5, -220) -> (-100, -220)
  line L889 (-100, -220) -> (-100, 220)
  dimension "d54" = 1.5
  dimension "d55" = 1.5
  constraint coincident L714.end L715.start
  constraint coincident L882 L884.end
  constraint perpendicular L882 L884
  constraint perpendicular L884 L885
  constraint coincident L880 L886.end
  constraint perpendicular L880 L886
  constraint coincident L244.end L245.start
  constraint coincident L880 L887.end
  constraint perpendicular L880 L887
  constraint perpendicular L887 L888
  constraint coincident L882 L889.end
  constraint perpendicular L882 L889
  measures "d54" distance of L884.end L885.end
  measures "d55" distance of L887.end L888.end
extrude "Extrude10" add sketch "Sketch7" along normal blind 3 contours L880 L882 L883 L889 | L880 L881 L882 L886 bodies 2
move_body "Move1" bodies 2 to x (1, 0, 0) y (0, 1, 0) z (0, 0, 1) at (0, 0, 3)
split "Split1" by plane through (0, 0, 0) normal (0, 1, 0) bodies 1 makes body 3 at (-102.8333, 113.8333, 13)
combine "Combine1" operation add target body 3 tool bodies 1
hidden bodies 2
named bodies: "Case side", "Lens side", "Case side (1)"
